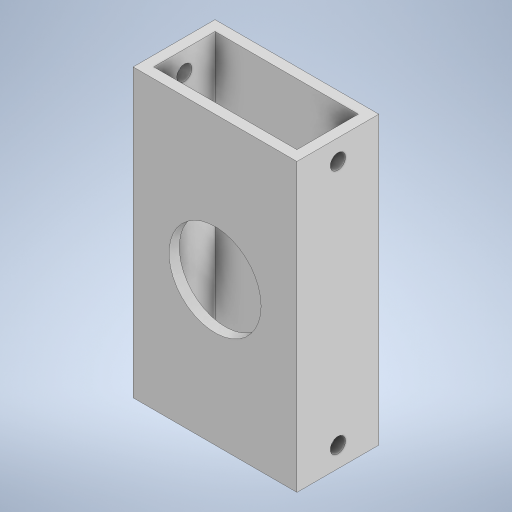
# Autodesk Inventor part: Bar
Saved by Autodesk Inventor 2023.1 (Build 271208000, 208)
## iProperties
Created: 2022-07-20
Part Number: Bar
Material: Generic
Document SubType Name: Modeling
Designer: Robotics
Density: 1 g/cm^3
Appearance: Default
Author: Robotics
Autodesk Inventor part; units mm, degrees
ref_plane "YZ Plane" through (0, 0, 0) normal (1, 0, 0) x (0, 1, 0)
ref_plane "XZ Plane" through (0, 0, 0) normal (0, 1, 0) x (-1, 0, 0)
ref_plane "XY Plane" through (0, 0, 0) normal (0, 0, 1) x (1, 0, 0)
sketch "Sketch3" plane through (0, 0, 0) normal (0, 1, 0) x (-1, 0, 0)
  line L0 (0, 0) -> (50.8, 0)
  line L1 (50.8, 0) -> (50.8, -25.4)
  line L2 (50.8, -25.4) -> (0, -25.4)
  line L3 (0, 0) -> (0, -25.4)
  dimension "d9" = 50.8
  dimension "d10" = 25.4
  dimension "d11" = 50.8
  constraints: 8 end point, 2 perpendicular, 1 horizontal
  measures "d9" distance of L0.start L0.end
  measures "d10" distance of L0.end L1.end
  measures "d11" distance of L1.end L2.end
extrude "Extrusion3" add sketch "Sketch3" along normal blind 88.9
sketch "Sketch4" plane through (0, 88.9, 0) normal (0, 1, 0) x (1, 0, 0)
  line L0 (0, 25.4) -> (-50.8, 25.4) projected
  line L1 (-50.8, 25.4) -> (-50.8, 0) projected
  line L2 (-50.8, 0) -> (0, 0) projected
  line L3 (0, 0) -> (0, 25.4) projected
  line L4 (-47.625, 22.225) -> (-3.175, 22.225)
  line L5 (-3.175, 22.225) -> (-3.175, 3.175)
  line L6 (-3.175, 3.175) -> (-47.625, 3.175)
  line L7 (-47.625, 3.175) -> (-47.625, 22.225)
  dimension "d14" = 3.175
  constraints: 8 end point, 3 other
  measures "d14" distance between parallel lines of L0 L4
extrude "Extrusion4" cut sketch "Sketch4" against normal blind 88.9 contours L4 L5 L6 L7
sketch "Sketch5" plane through (-50.8, 0, 0) normal (0, 0, 1) x (1, 0, 0)
  line L0 (0, 0) -> (0, 88.9) projected
  line L1 (0, 0) -> (25.4, 0)
  line L2 (0, 0) -> (50.8, 0) projected
  line L3 (25.4, 0) -> (25.4, 44.45)
  circle A0 centre (25.4, 44.45) radius 14.2875
  dimension "d17" = 25.4
  dimension "d18" = 44.45
  dimension "d19" = 28.575
  constraints: 4 end point, 1 centre point, 1 coincident, 1 midpoint, 1 perpendicular
  measures "d17" distance of L0.start L1.end
  measures "d18" distance of L1.end L3.end
  measures "d19" diameter of A0
extrude "Extrusion5" cut sketch "Sketch5" against normal blind 3.175
sketch "Sketch6" plane through (0, 0, 0) normal (1, 0, 0) x (0, 0, -1)
  line L0 (0, 0) -> (25.4, 0) projected
  line L1 (0, 0) -> (12.7, 0)
  line L2 (12.7, 0) -> (12.7, 6.35)
  circle A0 centre (12.7, 6.35) radius 2.3813
  line L3 (25.4, 0) -> (25.4, 88.9) projected
  line L4 (12.7, 6.35) -> (12.7, 82.55)
  circle A1 centre (12.7, 82.55) radius 2.3813
  dimension "d22" = 12.7
  dimension "d23" = 6.35
  dimension "d24" = 4.7625
  dimension "d26" = 76.2
  dimension "d27" = 4.7625
  constraints: 6 end point, 2 centre point, 2 coincident, 1 midpoint, 1 perpendicular, 1 vertical
  measures "d22" distance of L0.start L1.end
  measures "d23" distance of L1.end L2.end
  measures "d24" diameter of A0
  measures "d26" distance of L4.start L4.end
  measures "d27" diameter of A1
extrude "Extrusion6" cut sketch "Sketch6" against normal up to surface (50.8 mm away)
body "Solid2"
